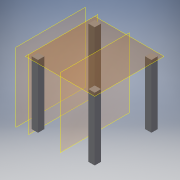
# Autodesk Inventor part: VeryBasicFrame
Saved by Autodesk Inventor 2016 SP1 (Build 200210100, 210)
## iProperties
Created: 2016-01-21
Part Number: VeryBasicFrame
Material: Generic
Document SubType Name: Modeling
Designer: steele
Density: 1 g/cm^3
Appearance: Default
Author: steele
Autodesk Inventor part; units mm, degrees
ref_plane "XY Plane" through (0, 0, 0) normal (0, 0, 1) x (1, 0, 0)
sketch "Sketch2" plane through (0, 0, 0) normal (0, 1, 0) x (-1, 0, 0)
  line L0 (127, 127) -> (101.6, 127)
  line L1 (101.6, 127) -> (101.6, 101.6)
  line L2 (101.6, 101.6) -> (127, 101.6)
  line L3 (127, 101.6) -> (127, 127)
  line L4 (101.6, 0) -> (-116.8124, 0) construction
  line L5 (0, 219.6692) -> (0, -132.8134) construction
  line L6 (127, -127) -> (101.6, -127)
  line L7 (101.6, -127) -> (101.6, -101.6)
  line L8 (101.6, -101.6) -> (127, -101.6)
  line L9 (127, -101.6) -> (127, -127)
  line L10 (-127, 127) -> (-101.6, 127)
  line L11 (-101.6, 127) -> (-101.6, 101.6)
  line L12 (-101.6, 101.6) -> (-127, 101.6)
  line L13 (-127, 101.6) -> (-127, 127)
  line L14 (-127, -127) -> (-101.6, -127)
  line L15 (-127, -101.6) -> (-127, -127)
  line L16 (-101.6, -101.6) -> (-127, -101.6)
  line L17 (-101.6, -127) -> (-101.6, -101.6)
  point P0 (0, 0)
  dimension "d1" = 25.4
  dimension "d2" = 101.6
  dimension "d3" = 101.6
  constraints: 36 end point, 12 symmetric about line, 2 horizontal, 2 parallel, 2 perpendicular, 1 vertical
  measures "d1" distance of L2.end L0.start
  measures "d2" distance from line of point (0, 0) L1
  measures "d3" distance from line of point (0, 0) L2
extrude "Extrusion1" add sketch "Sketch2" along normal blind 254
ref_plane "Work Plane1" through (-127, 254, 101.6) normal (0, 1, 0) x (-1, 0, 0)
ref_plane "Work Plane3" through (-177.8, 254, -101.6) normal (1, 0, 0) x (0, 1, 0)
ref_plane "Work Plane2" through (-127, 254, -101.6) normal (1, 0, 0) x (0, 1, 0)
body "Solid1"
